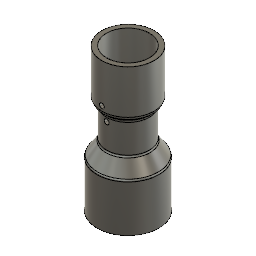
mass_airflow_tube (Autodesk Fusion 360 design; units mm, degrees)
Autodesk Fusion 360 part; units mm, degrees
sketch "Skizze1" plane through (0, 0, 0) normal (1, 0, 0) x (0, 0, -1)
  line L0 (-13, 0) -> (-13, 19)
  line L1 (-11.18, 17.291) -> (-11.18, 0)
  line L2 (-11.18, 0) -> (-13, 0)
  line L3 (0, 0) -> (-7.615, 0)
  line L4 (-7.615, 0) -> (-6.5, 0)
  line L5 (-7.615, 0) -> (-7.615, 17)
  line L6 (-7.615, 17) -> (-11.18, 17)
  line L7 (-6.5, 0) -> (-6.5, 20)
  line L8 (0, 0) -> (0, 53.458)
  line L9 (-6.5, 20) -> (-5, 35)
  line L10 (-11, 60) -> (-11, 43)
  line L11 (-13, 19) -> (-13, 19.5458)
  line L12 (-11, 60) -> (-9, 60)
  line L13 (-9, 60) -> (-9, 42)
  arc A0 (-5, 39) -> (-8, 42) centre (-8.5, 38.5) ccw
  line L14 (-9, 42) -> (-8, 42)
  line L15 (-5, 39) -> (-5, 35)
  line L16 (-12.7481, 20.3779) -> (-11, 23)
  line L17 (-11, 23) -> (-9.2519, 25.6221)
  line L18 (-9, 26.4542) -> (-9, 37)
  line L19 (-11, 43) -> (-11, 41.6213)
  line L20 (-10.5607, 40.5607) -> (-9.4393, 39.4393)
  line L21 (-9, 38.3787) -> (-9, 37)
  arc A1 (-11, 41.6213) -> (-10.5607, 40.5607) centre (-9.5, 41.6213) ccw
  arc A2 (-9, 38.3787) -> (-9.4393, 39.4393) centre (-10.5, 38.3787) ccw
  arc A3 (-9.2519, 25.6221) -> (-9, 26.4542) centre (-10.5, 26.4542) ccw
  arc A4 (-12.7481, 20.3779) -> (-13, 19.5458) centre (-11.5, 19.5458) ccw
  dimension "d3" = 7.615
  dimension "d4" = 1.115
  dimension "d7" = 1.5
  constraint vertical L0
  constraint perpendicular L0 L2
  constraint coincident L3.start L8.start
  constraint parallel L3 L4
  constraint perpendicular L3 L5
  constraint coincident L1 L6.end
  constraint perpendicular L1 L6
  constraint perpendicular L4 L7
  constraint perpendicular L3 L8
  constraint parallel L8 L10
  constraint parallel L0 L11
  constraint perpendicular L10 L12
  constraint perpendicular L12 L13
  constraint perpendicular L13 L14
  constraint perpendicular L14 L15
  constraint parallel L16 L17
  constraint parallel L11 L18
  constraint parallel L10 L19
  constraint parallel L18 L21
  constraint tangent L19 A1
  constraint tangent L20 A1
  constraint tangent L20 A2
  constraint tangent L21 A2
  constraint equal A1 A2
  constraint tangent L17 A3
  constraint tangent L18 A3
  constraint equal A1 A3
  constraint tangent L16 A4
  constraint tangent L11 A4
  constraint equal A1 A4
  measures "d3" distance of L3.start L3.end
  measures "d4" distance of L3.end L4.end
  measures "d7" radius of A1
revolve "Drehen1" add sketch "Skizze1" angle 360 about axis through (0, 0, 0) along (0, 1, 0)
hole "Bohrung1" at (0, 36.7372, 9) direction (0, 0, -1) diameter 2 depth 9 tip angle 118
hole "Bohrung2" at (0, 43.5811, 11) direction (0, 0, -1) diameter 2 depth 9 tip angle 118
